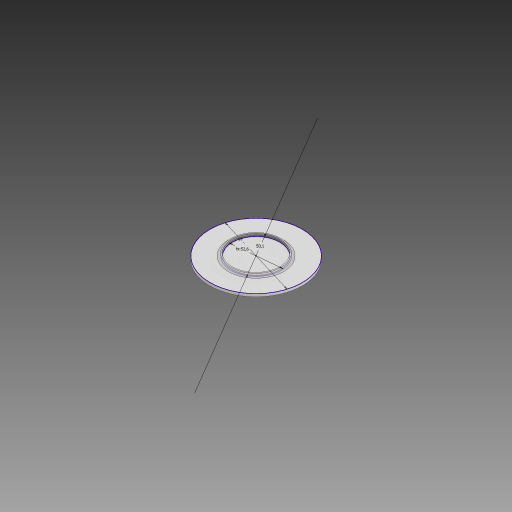
# Autodesk Inventor part: навес над зеркалом
Saved by Autodesk Inventor 2023 (Build 270158000, 158)
## iProperties
Created: 2025-04-21
Part Number: навес над зеркалом
Material: Типовые
Document SubType Name: Modeling
Designer: Ivan
Density: 1 g/cm^3
Appearance: По умолчанию
Author: Ivan
Autodesk Inventor part; units mm, degrees
ref_plane "YZ Plane" through (0, 0, 0) normal (1, 0, 0) x (0, 1, 0)
ref_plane "XZ Plane" through (0, 0, 0) normal (0, 1, 0) x (-1, 0, 0)
ref_plane "XY Plane" through (0, 0, 0) normal (0, 0, 1) x (1, 0, 0)
sketch "Эскиз1" plane through (0, 0, 0) normal (0, 1, 0) x (-1, 0, 0)
  circle A0 centre (0, 0) radius 25.05
  circle A1 centre (0, 0) radius 48.5
  circle A2 centre (0, 0) radius 26.3
  dimension "d1" = 50.1
  dimension "d2" = 97
  dimension "d3" = 52.6
  constraints: 3 centre point, 3 coincident
  measures "d1" diameter of A0
  measures "d2" diameter of A1
  measures "d3" diameter of A2
extrude "Выдавливание1" add sketch "Эскиз1" against normal blind 3 contours A0 | A1 | A2
extrude "Выдавливание2" add sketch "Эскиз1" along normal blind 2.6 contours A2
sketch "Эскиз2" plane through (0, -3, 0) normal (0, -1, 0) x (1, 0, 0)
  point P0 (0, 0)
hole "Отверстие1" at (0, -3, 0) direction (0, 1, 0) diameter 50 depth 1
chamfer "Фаска1" distance 2.6 angle 45 1 edges at (26.3, 0, 0)
